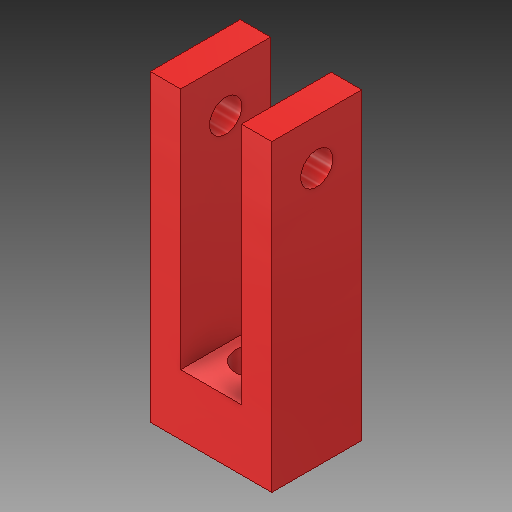
# Autodesk Inventor part: AngleBracketAttachementForDartActuator
Saved by Autodesk Inventor 2017 SP1 (Build 210196100, 196)
## iProperties
Created: 2016-06-07
Part Number: AngleBracketAttachementForDartActuator
Material: Generic
Document SubType Name: Modeling
Designer: steele
Density: 1 g/cm^3
Appearance: Light Red
Author: steele
Autodesk Inventor part; units mm, degrees
ref_plane "YZ Plane" through (0, 0, 0) normal (1, 0, 0) x (0, 1, 0)
ref_plane "XZ Plane" through (0, 0, 0) normal (0, 1, 0) x (-1, 0, 0)
ref_plane "XY Plane" through (0, 0, 0) normal (0, 0, 1) x (1, 0, 0)
sketch "Sketch7" plane through (0, 0, 0) normal (0, 1, 0) x (-1, 0, 0)
  line L0 (12.7, 9.398) -> (-12.7, 9.398)
  line L1 (-12.7, 9.398) -> (-12.7, -9.398)
  line L2 (-12.7, -9.398) -> (12.7, -9.398)
  line L3 (12.7, -9.398) -> (12.7, 9.398)
  line L4 (12.7, 9.398) -> (-12.7, -9.398) construction
  line L5 (-12.7, 9.398) -> (12.7, -9.398) construction
  point P0 (0, 0)
  dimension "d53" = 18.796
  dimension "d54" = 25.4
  constraints: 12 end point, 2 midpoint, 2 parallel, 1 horizontal, 1 perpendicular
  measures "d53" distance of L2.end L0.start
  measures "d54" distance of L1.end L2.end
extrude "Extrusion4" add sketch "Sketch7" along normal blind 63.5
sketch "Sketch8" plane through (0, 0, 0) normal (0, -1, 0) x (1, 0, 0)
  point P0 (0, 0)
  point P1 (0, 0)
  constraints: 1 coincident
hole "Hole7" at (0, 0, 0) direction (0, 1, 0) diameter 8.4328 depth 12.7 clearance for "Flat Head Machine Screw (82)" size "5/16" standard "Ansi Unified Screw Threads"
sketch "Sketch11" plane through (-12.7, 0, 9.398) normal (0, 0, 1) x (1, 0, 0)
  line L0 (12.7, 0) -> (12.7, 63.5) construction
  line L1 (0, 63.5) -> (25.4, 63.5) construction
  line L2 (19.05, 12.7) -> (19.05, 63.5)
  line L3 (19.05, 63.5) -> (6.35, 63.5)
  line L4 (6.35, 63.5) -> (6.35, 12.7)
  line L5 (6.35, 12.7) -> (19.05, 12.7)
  line L6 (19.05, 12.7) -> (6.35, 63.5) construction
  line L7 (19.05, 63.5) -> (6.35, 12.7) construction
  line L8 (0, 0) -> (25.4, 0) projected
  point P0 (12.7, 38.1)
  dimension "d85" = 12.7
  dimension "d86" = 50.8
  dimension "d87" = 12.7
  constraints: 14 end point, 3 midpoint, 2 parallel, 1 perpendicular, 1 point on line
  measures "d85" distance between parallel lines of L8 L5
  measures "d86" distance of L3.end L4.end
  measures "d87" distance of L4.end L2.start
extrude "Extrusion5" cut sketch "Sketch11" against normal through all
sketch "Sketch13" plane through (12.7, 0, 9.398) normal (1, 0, 0) x (0, 0, -1)
  line L0 (18.796, 63.5) -> (0, 63.5) construction
  line L1 (9.398, 63.5) -> (9.398, 0) construction
  point P0 (9.398, 53.975)
  dimension "d97" = 9.525
  constraints: 2 end point, 1 midpoint, 1 point on line, 1 vertical
  measures "d97" distance from line of point (9.398, 53.975) L0
hole "Hole10" at (12.7, 53.975, 0) direction (-1, 0, 0) diameter 6.7564 end through all clearance for "Flat Head Machine Screw (82)" size "1/4" standard "Ansi Unified Screw Threads"
body "Solid3"
